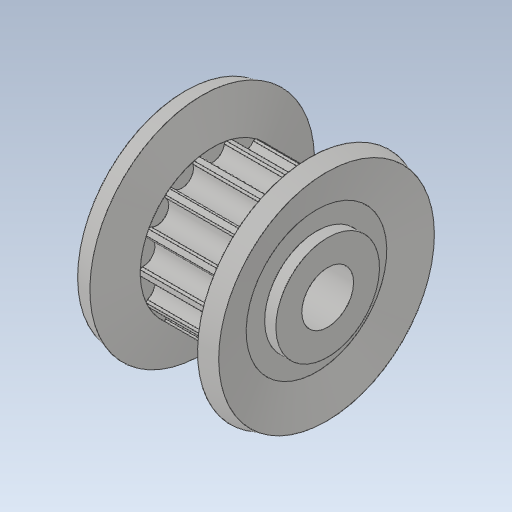
# Autodesk Inventor part: GPA14GT2040-A-H3_b
Saved by Autodesk Inventor 2024 (Build 280153000, 153)
## iProperties
Created: 2023-09-30
Part Number: GPA14GT2040-A-H3_b
Material: Generic
Catalog Web Link: www.cadenas.de
Description: GPA_GT2040, GPA_GT2060, GPA_GT2090, KGPA_GT2040, KGPA_GT2060, KGPA_GT2090, KGPK_GT2040, KGPK_GT2060, KGPK_GT2090_body-High Torque Timing Pulleys 2GT Type
Vendor: MISUMI
Document SubType Name: Modeling
Designer: psAdmin
Manufacturer: MISUMI
Mass: 0.459591 g
Surface Area: 7.80361 cm^2
Volume: 0.459591 cm^3
Density: 1 g/cm^3
Appearance: PSOLRGB-175-175-175
Category: PARTsolutions
Company: MISUMI
PSOL_IDENT_0: {$CADENAS_DATA/23d-libs/misumi/metric/51_timing_pulleys/gpa__gt2/gpa_gt2.prj},476 {VTYP=3D},{NB=GPA1
PSOL_IDENT_1: 4GT2040-A-H3_b},{LINA=GPA14GT2040-A-H3},{NN=GPA_GT2040, GPA_GT2060, GPA_GT2090, KGPA_GT2040, KGPA_GT
PSOL_IDENT_2: 2060, KGPA_GT2090, KGPK_GT2040, KGPK_GT2060, KGPK_GT2090_body},{DATE=25.04.2022 01:22:58},{GEOMDATE=
PSOL_IDENT_3: 22.12.2021 00:45:33},{VERSION=},{LINEID=30},{WBVAR=MAT,ST,TNW,PS,SBS,DD,Z,J,Q,R,S,T,ALT1,ALT2,M,QSC,
PSOL_IDENT_4: QFC,QTC,ALT3,K,KSC,KFC,KTC,ALT4,ZM,ZSC,ZFC,ZTC,ALT5,BC,ALT6,ALT7,ALT8,FC,ALT13,BN},{WBNUMERIC=DD,Z,J
PSOL_IDENT_5: ,Q,R,S,T,QSC,QFC,QTC,K,KSC,KFC,KTC,ZSC,ZFC,ZTC,BC,FC,BN}  {NB=GPA14GT2040-A-H3_b},{LINA=GPA14GT2040-
PSOL_IDENT_6: A-H3},{KT=DUMMY},{PN=GPA14GT2040-A-H3},{TYPE=GPA},{MAT=AA},{ST=CA},{NT=14},{TNW=GT2040},{BW=0},{A=5.
PSOL_IDENT_7: 0},{W=8.3},{L=16.0},{PS=A},{PSA= 'A' },{SBS=H},{SBSALG= 'H','Round Hole' },{DD=3.00},{DDALG=[3:3/1]}
PSOL_IDENT_8: ,{DDHA=[3:3/1]},{DDHB=},{DDPA=},{DDPB=},{DDNA=},{DDNB=},{DDNKA=0},{DDNKB=0},{DDVA=},{DDVFB=},{DDYA=}
PSOL_IDENT_9: ,{Z=0},{ZALG=0},{ZMIN=5},{ZAMAX=0},{ZBMAX=0},{J=0.0},{JALG=0},{JMAX=6.3},{Q=0},{R=0},{QRALG=0},{QRMI
PSOL_IDENT_10: N=5},{QRMAX=0},{S=0.0},{SALG=0},{SMAX=2.300},{T=0.0},{TALG=0},{TMAX=5.000},{PD=8.91},{OD=8.40},{D=0}
PSOL_IDENT_11: ,{DE=6},{DDZ=3},{F=13},{E=6},{BB=0},{TT=0},{M1=0},{AC=-},{ALT1=},{ALT1A= '','Not applicable' },{ANG=
PSOL_IDENT_12: 128.571429},{ALT2=},{ALT2A= '','Not applicable' },{M=N/A},{MALG= 'N/A' },{MM=0.000},{MPHD=0.000},{MA=
PSOL_IDENT_13: 'N/A' },{MSA= 'N/A' },{QSC=0.0},{QSCA=0},{QFC=0.0},{QFCA=0},{QTC=0.0},{QTCA=0},{QPCDMIN=7},{QPCDMIN
PSOL_IDENT_14: ALG=7},{QPCDMAX=2},{ALT2PN=},{ALT3=},{ALT3A= '','Not applicable' },{K=0.0},{KA=0},{KAMIN=4},{KAMAX=0
PSOL_IDENT_15: },{KSMAX=0},{KSC=0.0},{KSCA=0},{KFC=0.0},{KFCA=0},{KTC=0.0},{KTCA=0},{KSCMIN=7.000},{KPCDMIN=7.000},
PSOL_IDENT_16: {KPCDMINALG=11.000},{KPCDMAX=2.000},{ALT3PN=},{ALT4=},{ALT4ALG= '','Not applicable' },{ALT4MIN=13.50
PSOL_IDENT_17: 0},{ALT4MAX=-4.500},{ZM=N/A},{ZMALG= 'N/A' },{ZMFTALG= 'N/A' },{ZMSALG= 'N/A' },{ZMDD1=0.0},{ZMDD2=0
PSOL_IDENT_18: .0},{ZMHH=0.0},{ZSC=0.0},{ZSCALG=[0]},{ZFC=0.0},{ZFCALG=[0]},{ZTC=0.0},{ZTCALG=[0]},{ZPCDMIN=0.000},
PSOL_IDENT_19: {ZPCDMINALG=0.000},{ZPCDMAX=2.000},{ALT4PN=},{ALT5=},{ALT5ALG= '','Not applicable' },{ALT5PN=},{BC=0
PSOL_IDENT_20: .0},{BCALG=0},{BCMIN=3.000},{BCMAX=7.700},{ALT6=},{ALT7=},{ALT7ALG= '','w/o Flange Attached on One S
PSOL_IDENT_21: ide Only','-RFC','with RFC (Flange Attached on The Boss Side Only)','-LFC','with LFC (Flange Attache
PSOL_IDENT_22: d on The Opposite Side Only)' },{ALT8=},{ALT8ALG='','w/o FC (Flange Cut)','-FC','with FC (Flange Cut
PSOL_IDENT_23: )'},{ALT8PN=},{FC=0.0},{FCA=0},{ODAINT=11.500},{FCMIN=9.5},{FCMAX=11},{WLBC=8.3},{SL=1.5},{SL2=4.5},
PSOL_IDENT_24: {KTT=1.5},{KYY=2.7},{TAP=0},{MATALG= 'AA','Aluminum Alloy 2000 series' , '6000','6000 Series Aluminu
PSOL_IDENT_25: m Alloy' },{STALG= 'CA','Clear Anodize' },{ALT13=},{BN=0.000},{BNMIN=8.200},{BNMAX=17.700},{ALT13ALG=
PSOL_IDENT_26: '','Not applicable' },{BNALG=0},{BNPN=}
NB: GPA14GT2040-A-H3_b
NN: GPA_GT2040, GPA_GT2060, GPA_GT2090, KGPA_GT2040, KGPA_GT2060, KGPA_GT2090, KGPK_GT2040, KGPK_GT2060, KGPK_GT2090_body
NT: 14
NBSYN: $PN._b
LINA: GPA14GT2040-A-H3
CATALOG: Misumi
PN: GPA14GT2040-A-H3
MAT: Aluminum Alloy 2000 series
ST: Clear Anodize
TNW: GT2040
A: 5
W: 8.3
L: 16
PS: A
SBS: Round Hole
DD: 3
Z: 0
J: 0
Q: 0
R: 0
S: 0
T: 0
PD: 8.91
OD: 8.4
D: 0
F: 13
E: 6
AC: -
ALT1: Not applicable
ALT2: Not applicable
M: N/A
QSC: 0
QFC: 0
QTC: 0
ALT3: Not applicable
K: 0
KSC: 0
KFC: 0
KTC: 0
ALT4: Not applicable
ZM: N/A
ZMDD1: 0
ZMDD2: 0
ZMHH: 0
ZSC: 0
ZFC: 0
ZTC: 0
ALT5: Not applicable
BC: 0
ALT6: w/o Flange not Attached
ALT7: w/o Flange Attached on One Side Only
ALT8: w/o FC (Flange Cut)
FC: 0
ALT13: Not applicable
BN: 0
SUPPLIER: MISUMI
ARTICLENO: GPA14GT2040-A-H3_b
BOMINFO: GPA14GT2040-A-H3
CREATOR: CADENAS GmbH
Title: GPA14GT2040-A-H3
Author: Cadenas PARTsolutions
Comments: High Torque Timing Pulleys 2GT Type
Autodesk Inventor part; units mm, degrees
note: some values were not read from the file. Chosen so that the rebuilt part matches the saved one: pattern direction of "Circular Pattern1".
ref_plane "YZ Plane" through (0, 0, 0) normal (1, 0, 0) x (0, 1, 0)
ref_plane "XZ Plane" through (0, 0, 0) normal (0, 1, 0) x (-1, 0, 0)
ref_plane "XY Plane" through (0, 0, 0) normal (0, 0, 1) x (1, 0, 0)
sketch "Sketch_16" plane through (0, 0, 0) normal (0, 0, 1) x (1, 0, 0)
  line L0 (4.15, 0) -> (-4.15, 0)
  line L1 (-4.15, 0) -> (-4.15, 3)
  line L2 (-4.15, 3) -> (-2.5, 3)
  line L3 (-2.5, 3) -> (-2.5, 4.2)
  line L4 (-2.5, 4.2) -> (2.5, 4.2)
  line L5 (2.5, 4.2) -> (2.5, 3)
  line L6 (2.5, 3) -> (4.15, 3)
  line L7 (4.15, 3) -> (4.15, 0)
  line L8 (4.15, 0) -> (-4.15, 0)
  constraints: 18 end point
revolve "Revolution1" add sketch "Sketch_16" angle 360 about axis through (4.15, 0, 0) along (1, 0, 0)
sketch "Sketch_18" plane through (0, 0, 0) normal (1, 0, 0) x (0, 1, 0)
  line L0 (4.3536, 0.9449) -> (4.1064, 0.8912)
  line L1 (4.1064, 0.8912) -> (4.1241, 0.8003)
  arc A0 (4.03, 0.6681) -> (4.1241, 0.8003) centre (4.0141, 0.779) ccw
  arc A1 (4.03, 0.6681) -> (4.03, -0.6681) centre (4.126, 0) ccw
  arc A2 (4.1241, -0.8003) -> (4.03, -0.6681) centre (4.0141, -0.779) ccw
  line L2 (4.1241, -0.8003) -> (4.1064, -0.8912)
  line L3 (4.1064, -0.8912) -> (4.3536, -0.9449)
  arc A3 (4.3536, -0.9449) -> (4.3536, 0.9449) centre (0, 0) ccw
  constraints: 8 end point, 8 point on circle, 4 centre point
extrude "Extrusion1" cut sketch "Sketch_18" along normal mid plane 5
pattern_circular "Circular Pattern1" count 14 over 360 about axis through (0, 0, 0) along (1, 0, 0) of "Extrusion1"
sketch "Sketch_20" plane through (0, 0, 0) normal (0, 0, 1) x (1, 0, 0)
  line L0 (50, 0) -> (-50, 0)
  line L1 (2.5, 4.2) -> (2.5, 3)
  line L2 (2.5, 3) -> (3.5, 3)
  line L3 (3.5, 3) -> (3.5, 4.0683)
  line L4 (3.5, 4.0683) -> (4.0822, 6.2412)
  line L5 (4.0822, 6.2412) -> (3.1163, 6.5)
  line L6 (3.1163, 6.5) -> (2.5, 4.2)
  constraints: 14 end point
revolve "Revolution2" add sketch "Sketch_20" angle 360 about axis through (50, 0, 0) along (1, 0, 0)
sketch "Sketch_21" plane through (0, 0, 0) normal (0, 0, 1) x (1, 0, 0)
  line L0 (50, 0) -> (-50, 0)
  line L1 (-4.0822, 6.2412) -> (-3.5, 4.0683)
  line L2 (-3.5, 4.0683) -> (-3.5, 3)
  line L3 (-3.5, 3) -> (-2.5, 3)
  line L4 (-2.5, 3) -> (-2.5, 4.2)
  line L5 (-2.5, 4.2) -> (-3.1163, 6.5)
  line L6 (-3.1163, 6.5) -> (-4.0822, 6.2412)
  constraints: 14 end point
revolve "Revolution3" add sketch "Sketch_21" angle 360 about axis through (50, 0, 0) along (1, 0, 0)
sketch "Sketch5" plane through (4.15, 0, 0) normal (1, 0, 0) x (0, 0, -1)
  point P0 (0, 0)
hole "Hole1" at (4.15, 0, 0) direction (-1, 0, 0) diameter 3 depth 8.3
body "Solid1"
